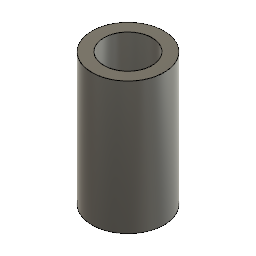
spacer_for_rpi_mount_11mm (Autodesk Fusion 360 design; units mm, degrees)
Autodesk Fusion 360 part; units mm, degrees
sketch "スケッチ1" plane through (0, 0, 0) normal (0, 1, 0) x (1, 0, 0)
  circle A0 centre (0, 0) radius 1.3
  circle A1 centre (0, 0) radius 2.5
  circle A2 centre (0, 0) radius 1.5
  dimension "d1" = 2.6
  constraint coincident A0.centre A1.centre
  measures "d1" diameter of A0
extrude "押し出し2" add sketch "スケッチ1" along normal blind 11 contours A1 makes body 1
extrude "押し出し1" add sketch "スケッチ1" along normal blind 11 separate body contours A1 | A2 makes body 2
sketch "スケッチ2" plane through (0, 0, 0) normal (0, 1, 0) x (1, 0, 0)
  circle A0 centre (0, 0) radius 2
  circle A1 centre (0, 0) radius 3
  constraint coincident A0.centre A1.centre
extrude "押し出し3" add sketch "スケッチ2" along normal blind 11 separate body makes body 3
hidden bodies 1 2
